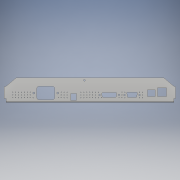
# Autodesk Inventor part: BLACHA OBUDOWY TYLNEJ MONITORA
Saved by Autodesk Inventor 2017 SP1 (Build 210196100, 196)
## iProperties
Created: 2021-02-21
Part Number: BLACHA OBUDOWY TYLNEJ MONITORA
Material: Generic
Document SubType Name: Modeling
Designer: Napoleon
Density: 1 g/cm^3
Appearance: Default
Mass: 13.3476 g
Surface Area: 281.222 cm^2
Volume: 13.3476 cm^3
Author: Napoleon
Autodesk Inventor part; units mm, degrees
ref_plane "YZ Plane" through (0, 0, 0) normal (1, 0, 0) x (0, 1, 0)
ref_plane "Płaszczyzna konstrukcyjna1" through (0, 0, 0) normal (0, 0, 1) x (1, 0, 0)
ref_plane "Płaszczyzna konstrukcyjna11" through (0, 0, 0) normal (0, 0, -1) x (-1, 0, 0)
sketch "Szkic3" plane through (0, 0, 0) normal (0, 0, -1) x (-1, 0, 0)
  line L0 (203.9997, -35) -> (-75.9997, -35) projected
  line L1 (203.9997, -35) -> (-75.9997, -35)
  line L2 (-75.9997, -35) -> (-75.9997, -34)
  line L3 (-75.9997, -34) -> (203.9997, -34)
  line L4 (203.9997, -34) -> (203.9997, -35)
  dimension "d23" = 1
  constraints: 8 end point, 2 parallel, 1 horizontal, 1 perpendicular
  measures "d23" distance of L1.end L2.end
extrude "Wyciągnięcie proste3" add sketch "Szkic3" along normal blind 15
sketch "Szkic1" plane through (0, 0, 0) normal (0, 0, 1) x (1, 0, 0)
  line L0 (75.9997, -29) -> (79, -29)
  line L1 (79, -29) -> (79, -9.3813)
  line L2 (79, -9.3813) -> (75.9997, -8.5)
  line L3 (75.9997, -8.5) -> (59.2898, 5.5714)
  line L4 (59.2898, 5.5714) -> (-187.2898, 5.5714)
  line L5 (-187.2898, 5.5714) -> (-203.9997, -8.5)
  line L6 (-203.9997, -8.5) -> (-207, -9.3813)
  line L7 (-207, -29) -> (-207, -9.3813)
  line L8 (-207, -29) -> (-203.9997, -29)
  line L9 (-5.575, -26.25) -> (-5.575, -13.25)
  line L10 (-176.45, -11.176) -> (-191.7, -11.176)
  line L11 (-191.7, -11.176) -> (-191.7, -25.7107)
  line L12 (-41.3, -32) -> (-31.8, -32)
  line L13 (-31.8, -32) -> (-31.8, -20.5)
  line L14 (-31.8, -20.5) -> (-41.3, -20.5)
  line L15 (-41.3, -20.5) -> (-41.3, -32)
  circle A0 centre (-54.6, 1.5) radius 1.5
  line L16 (-0.575, -31.25) -> (20.175, -31.25)
  circle A1 centre (65.05, -22.9757) radius 0.625
  circle A2 centre (65.05, -18.4635) radius 0.625
  circle A3 centre (65.05, -27.4878) radius 0.625
  circle A4 centre (60.15, -22.9757) radius 0.625
  circle A5 centre (60.15, -18.4635) radius 0.625
  circle A6 centre (60.15, -27.4878) radius 0.625
  circle A7 centre (55.25, -22.9757) radius 0.625
  circle A8 centre (55.25, -18.4635) radius 0.625
  circle A9 centre (55.25, -27.4878) radius 0.625
  circle A10 centre (50.35, -22.9757) radius 0.625
  circle A11 centre (50.35, -18.4635) radius 0.625
  circle A12 centre (50.35, -27.4878) radius 0.625
  circle A13 centre (45.45, -22.9757) radius 0.625
  circle A14 centre (45.45, -18.4635) radius 0.625
  circle A15 centre (45.45, -27.4878) radius 0.625
  circle A16 centre (40.55, -22.9757) radius 0.625
  circle A17 centre (40.55, -18.4635) radius 0.625
  circle A18 centre (40.55, -27.4878) radius 0.625
  circle A19 centre (35.65, -22.9757) radius 0.625
  circle A20 centre (35.65, -18.4635) radius 0.625
  circle A21 centre (35.65, -27.4878) radius 0.625
  circle A22 centre (30.75, -27.4878) radius 0.625
  circle A23 centre (-11.15, -27.4878) radius 0.625
  circle A24 centre (-16.05, -22.9757) radius 0.625
  circle A25 centre (-16.05, -18.4635) radius 0.625
  circle A26 centre (-16.05, -27.4878) radius 0.625
  circle A27 centre (-20.95, -22.9757) radius 0.625
  circle A28 centre (-20.95, -18.4635) radius 0.625
  circle A29 centre (-20.95, -27.4878) radius 0.625
  circle A30 centre (-25.85, -22.9757) radius 0.625
  circle A31 centre (-25.85, -18.4635) radius 0.625
  circle A32 centre (-25.85, -27.4878) radius 0.625
  circle A33 centre (-48.75, -22.9757) radius 0.625
  circle A34 centre (-48.75, -18.4635) radius 0.625
  circle A35 centre (-48.75, -27.4878) radius 0.625
  circle A36 centre (-53.65, -22.9757) radius 0.625
  circle A37 centre (-53.65, -18.4635) radius 0.625
  circle A38 centre (-53.65, -27.4878) radius 0.625
  circle A39 centre (-58.55, -22.9757) radius 0.625
  circle A40 centre (-58.55, -18.4635) radius 0.625
  circle A41 centre (-58.55, -27.4878) radius 0.625
  circle A42 centre (-63.45, -22.9757) radius 0.625
  circle A43 centre (-63.45, -18.4635) radius 0.625
  circle A44 centre (-63.45, -27.4878) radius 0.625
  circle A45 centre (-68.35, -22.9757) radius 0.625
  circle A46 centre (-68.35, -18.4635) radius 0.625
  circle A47 centre (-68.35, -27.4878) radius 0.625
  line L17 (-203.9997, -29) -> (-203.9997, -35)
  line L18 (75.9997, -29) -> (75.9997, -35)
  line L19 (75.9997, -35) -> (-203.9997, -35)
  line L20 (-107.21, -19.1157) -> (-107.21, -18.8657)
  line L21 (-108.46, -20.1114) -> (-108.46, -23.9361)
  line L22 (-107.742, -25.7587) -> (-108.46, -23.9361)
  arc A48 (-107.21, -18.8657) -> (-108.46, -20.1114) centre (-107.2143, -20.1114) ccw
  arc A49 (-107.742, -25.7587) -> (-105.9103, -27.0857) centre (-105.7879, -24.989) ccw
  line L23 (-85.18, -19.1157) -> (-85.1757, -18.8657)
  line L24 (-83.93, -20.1114) -> (-83.93, -23.9361)
  line L25 (-84.648, -25.7587) -> (-83.93, -23.9361)
  arc A50 (-83.93, -20.1114) -> (-85.1757, -18.8657) centre (-85.1757, -20.1114) ccw
  arc A51 (-86.4797, -27.0857) -> (-84.648, -25.7587) centre (-86.6021, -24.989) ccw
  line L26 (-85.1757, -18.8657) -> (-107.21, -18.8657)
  line L27 (-105.9103, -27.0857) -> (-86.4797, -27.0857)
  circle A52 centre (-79.94, -22.9757) radius 1.4224
  circle A53 centre (-112.45, -22.9757) radius 1.4224
  circle A54 centre (-73.25, -27.4878) radius 0.625
  circle A55 centre (-78.15, -27.4878) radius 0.625
  circle A56 centre (-83.05, -27.4878) radius 0.625
  circle A57 centre (-112.45, -27.4878) radius 0.625
  circle A58 centre (-117.35, -27.4878) radius 0.625
  circle A59 centre (-122.25, -27.4878) radius 0.625
  circle A60 centre (-146.75, -27.4878) radius 0.625
  circle A61 centre (-151.65, -27.4878) radius 0.625
  line L28 (-160.3, -25.7107) -> (-172.45, -25.7107)
  line L29 (-176.45, -25.7107) -> (-191.7, -25.7107)
  line L30 (-176.45, -25.7107) -> (-176.45, -11.176)
  circle A62 centre (-73.25, -18.4635) radius 0.625
  circle A63 centre (-73.25, -22.9757) radius 0.625
  circle A64 centre (-117.35, -22.9757) radius 0.625
  circle A65 centre (-117.35, -18.4635) radius 0.625
  circle A66 centre (-151.65, -22.9757) radius 0.625
  circle A67 centre (-78.15, -18.4635) radius 0.625
  circle A68 centre (-122.2486, -18.4635) radius 0.625
  circle A69 centre (-121.7514, -22.9757) radius 1.4224
  circle A70 centre (-146.7514, -18.4635) radius 0.625
  circle A71 centre (-146.7514, -22.9757) radius 1.4224
  circle A72 centre (-151.65, -18.4648) radius 0.625
  line L31 (25.175, -26.25) -> (25.175, -13.25)
  line L32 (-0.575, -8.25) -> (20.175, -8.25)
  arc A73 (25.175, -13.25) -> (20.175, -8.25) centre (20.175, -13.25) ccw
  arc A74 (-0.575, -8.25) -> (-5.575, -13.25) centre (-0.575, -13.25) ccw
  arc A75 (-5.575, -26.25) -> (-0.575, -31.25) centre (-0.575, -26.25) ccw
  arc A76 (20.175, -31.25) -> (25.175, -26.25) centre (20.175, -26.25) ccw
  line L33 (-140.6225, -27.2951) -> (-127.8804, -27.2951)
  line L34 (-126.7087, -18.2951) -> (-141.7942, -18.2951)
  line L35 (-126.6016, -26.2292) -> (-125.4299, -19.8292)
  line L36 (-141.9012, -26.2292) -> (-143.0729, -19.8292)
  arc A77 (-125.4299, -19.8292) -> (-126.7087, -18.2951) centre (-126.7087, -19.5951) ccw
  arc A78 (-127.8804, -27.2951) -> (-126.6016, -26.2292) centre (-127.8804, -25.9951) ccw
  arc A79 (-141.7942, -18.2951) -> (-143.0729, -19.8292) centre (-141.7942, -19.5951) ccw
  arc A80 (-141.9012, -26.2292) -> (-140.6225, -27.2951) centre (-140.6225, -25.9951) ccw
  circle A81 centre (29.8, -19.75) radius 1.75
  circle A82 centre (-10.2, -19.75) radius 1.75
  line L37 (-160.3, -25.7107) -> (-160.075, -25.7107)
  line L38 (-160.075, -25.7107) -> (-160.075, -14.4607)
  line L39 (-172.45, -25.7107) -> (-172.675, -25.7107)
  line L40 (-172.675, -25.7107) -> (-172.675, -14.4607)
  line L41 (-160.075, -14.4607) -> (-172.675, -14.4607)
  point P0 (0, 0)
  point P1 (-5.575, -31.25)
  point P2 (25.175, -31.25)
  dimension "d21" = 6
  dimension "d22" = 6
  dimension "d97" = 4.625
  dimension "d98" = 11.5
  dimension "d103" = 0.225
  dimension "d104" = 11.25
  constraints: 84 end point, 83 centre point, 24 point on circle, 14 tangent, 5 horizontal, 5 perpendicular, 4 equal radius, 4 point on line, 3 parallel, 3 vertical
  measures "d21" distance of L8.end L17.end
  measures "d22" distance of L0.start L18.end
  measures "d97" distance from line of L31 A81.centre
  measures "d98" distance from line of L16 A81.centre
  measures "d103" distance of L28.start L37.end
  measures "d104" distance of L37.end L38.end
extrude "Wyciągnięcie proste18" add sketch "Szkic1" along normal blind 1
